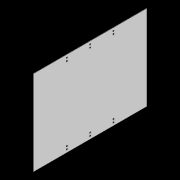
# Autodesk Inventor part: BottomV4
Saved by Autodesk Inventor 2022 (Build 260153000, 153)
## iProperties
Created: 2021-10-02
Part Number: BottomV4
Material: Generic
Document SubType Name: Modeling
Designer: timmy
Density: 1 g/cm^3
Appearance: Default
Author: timmy
Autodesk Inventor part; units mm, degrees
ref_plane "YZ Plane" through (0, 0, 0) normal (1, 0, 0) x (0, 1, 0)
ref_plane "XZ Plane" through (0, 0, 0) normal (0, 1, 0) x (-1, 0, 0)
ref_plane "XY Plane" through (0, 0, 0) normal (0, 0, 1) x (1, 0, 0)
sketch "Sketch1" plane through (0, 0, 0) normal (1, 0, 0) x (0, 1, 0)
  line L0 (0, 0) -> (381, 0)
  line L1 (381, 0) -> (381, -508)
  line L2 (381, -508) -> (0, -508)
  line L3 (0, -508) -> (0, 0)
  dimension "d0" = 381
  dimension "d1" = 508
  constraints: 8 end point, 2 parallel, 1 horizontal, 1 perpendicular
  measures "d0" distance of L1.end L2.end
  measures "d1" distance of L0.end L1.end
extrude "Extrusion1" add sketch "Sketch1" along normal blind 1.5875
sketch "Sketch3" plane through (0, 0, 0) normal (-1, 0, 0) x (0, 0, 1)
  line L0 (-508, 0) -> (-508, 381) projected
  line L1 (0, 0) -> (-508, 0) projected
  circle A0 centre (-358.14, 12.7) radius 3.302
  circle A1 centre (-358.14, 25.4) radius 3.302
  circle A2 centre (-358.14, 368.3) radius 3.302
  circle A3 centre (-358.14, 355.6) radius 3.302
  circle A4 centre (-149.86, 12.7) radius 3.302
  circle A5 centre (-149.86, 25.4) radius 3.302
  circle A6 centre (-149.86, 368.3) radius 3.302
  circle A7 centre (-149.86, 355.6) radius 3.302
  circle A8 centre (-254, 12.7) radius 3.302
  circle A9 centre (-254, 25.4) radius 3.302
  circle A10 centre (-254, 368.3) radius 3.302
  circle A11 centre (-254, 355.6) radius 3.302
  constraints: 12 centre point
extrude "Extrusion5" cut sketch "Sketch3" against normal up to surface (1.5875 mm away)
body "Solid1"
